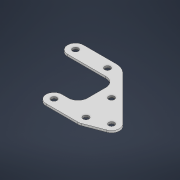
# Autodesk Inventor part: gusset-2-3.25-half
Saved by Autodesk Inventor 2021 (Build 250183000, 183)
## iProperties
Created: 2020-11-04
Part Number: gusset-2-3.25-half
Material: Generic
Document SubType Name: Modeling
Designer: Carlos Stewart
Density: 1 g/cm^3
Appearance: Default
Author: Carlos Stewart
Autodesk Inventor part; units mm, degrees
ref_plane "YZ Plane" through (0, 0, 0) normal (1, 0, 0) x (0, 1, 0)
ref_plane "XZ Plane" through (0, 0, 0) normal (0, 1, 0) x (-1, 0, 0)
ref_plane "XY Plane" through (0, 0, 0) normal (0, 0, 1) x (1, 0, 0)
sketch "Sketch1" plane through (0, 0, 0) normal (0, 1, 0) x (-1, 0, 0)
  line L0 (-37.8542, -1.1176) -> (-32.7742, -1.1176)
  line L1 (-7.3742, -30.9118) -> (-37.8542, -30.9118)
  line L2 (-45.4742, -23.2918) -> (-45.4742, -8.7376)
  arc A0 (-37.8542, -1.1176) -> (-45.4742, -8.7376) centre (-37.8542, -8.7376) ccw
  arc A1 (-45.4742, -23.2918) -> (-37.8542, -30.9118) centre (-37.8542, -23.2918) ccw
  circle A2 centre (-72.8662, -0.3634) radius 2.3114
  circle A3 centre (-54.9057, -18.324) radius 2.3114
  circle A4 centre (-58.1742, 5.2324) radius 2.3114
  circle A5 centre (-32.7742, 5.2324) radius 2.3114
  circle A6 centre (-32.7742, -37.2618) radius 2.3114
  circle A7 centre (-7.3742, -37.2618) radius 2.3114
  arc A8 (-75.1264, 5.5707) -> (-77.3564, -4.8536) centre (-72.8662, -0.3634) ccw
  arc A9 (-32.7742, -43.6118) -> (-31.4271, -43.4673) centre (-32.7742, -37.2618) ccw
  arc A10 (-7.3742, -43.6118) -> (-7.3742, -30.9118) centre (-7.3742, -37.2618) ccw
  arc A11 (-32.7742, -1.1176) -> (-32.7742, 11.5824) centre (-32.7742, 5.2324) ccw
  arc A12 (-58.1742, 11.5824) -> (-60.4344, 11.1665) centre (-58.1742, 5.2324) ccw
  line L3 (-32.7742, 11.5824) -> (-58.1742, 11.5824)
  line L4 (-75.1264, 5.5707) -> (-60.4344, 11.1665)
  line L5 (-77.3564, -4.8536) -> (-42.3179, -39.8921)
  line L6 (-33.3376, -43.6118) -> (-7.3742, -43.6118)
  arc A13 (-42.3179, -39.8921) -> (-33.3376, -43.6118) centre (-33.3376, -30.9118) ccw
  line L7 (-37.8542, -1.1176) -> (-32.7742, -1.1176)
  point P0 (0, 0)
  point P1 (-45.4742, -30.9118)
  dimension "d2" = 7.62
  dimension "d20" = 12.7
  dimension "d21" = 29.7942
  constraints: 17 point on circle, 16 end point, 14 centre point, 13 tangent, 5 coincident, 3 point on line, 2 horizontal, 1 equal radius, 1 parallel, 11 other
  measures "d2" radius of A0
  measures "d20" radius of A13
  measures "d21" distance between parallel lines of L0 L1
extrude "Extrusion1" add sketch "Sketch1" along normal blind 1.5875
body "Solid1"
